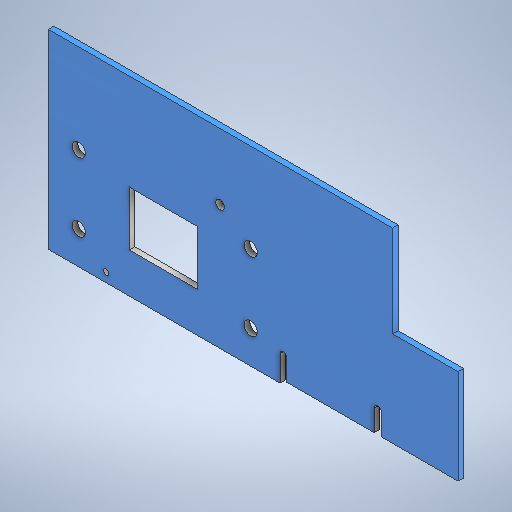
# Autodesk Inventor part: daughterboard
Saved by Autodesk Inventor 2025.1 (Build 291241000, 241)
## iProperties
Created: 2024-09-23
Part Number: daughterboard
Material: Generic
Document SubType Name: Modeling
Designer: PC
Density: 1 g/cm^3
Appearance: Default
Author: PC
Autodesk Inventor part; units mm, degrees
ref_plane "YZ Plane" through (0, 0, 0) normal (1, 0, 0) x (0, 1, 0)
ref_plane "XZ Plane" through (0, 0, 0) normal (0, 1, 0) x (-1, 0, 0)
ref_plane "XY Plane" through (0, 0, 0) normal (0, 0, 1) x (1, 0, 0)
sketch "Sketch1" plane through (0, 0, 0) normal (0, 0, 1) x (1, 0, 0)
  line L0 (0, 0) -> (125, 0)
  line L1 (125, 1.25) -> (125, 30.15)
  line L2 (105, 58.1) -> (0, 58.1)
  line L3 (0, 58.1) -> (0, 0)
  line L4 (105, 58.1) -> (105, 30.15)
  line L5 (105, 30.15) -> (125, 30.15)
  line L6 (24.7, 28.775) -> (45.44, 28.775)
  line L7 (45.44, 28.775) -> (45.44, 12.175)
  line L8 (45.44, 12.175) -> (24.7, 12.175)
  line L9 (24.7, 12.175) -> (24.7, 28.775)
  circle A0 centre (9.3, 10) radius 2
  circle A1 centre (61.75, 10) radius 2
  circle A2 centre (9.3, 30.95) radius 2
  circle A3 centre (61.75, 30.95) radius 2
  line L10 (9.3, 30.95) -> (9.3, 10) construction
  line L11 (9.3, 10) -> (61.75, 10) construction
  line L12 (70.7, 0) -> (70.7, 1.25)
  arc A4 (72.7, 7.8) -> (70.7, 7.8) centre (71.7, 7.8) ccw
  line L13 (70.7, 7.8) -> (70.7, 1.25)
  line L14 (72.7, 7.8) -> (72.7, 1.25)
  arc A5 (101.6, 7.8) -> (99.4, 7.8) centre (100.5, 7.8) ccw
  line L15 (99.4, 7.8) -> (99.4, 1.25)
  line L16 (101.6, 7.8) -> (101.6, 1.25)
  line L17 (72.7, 1.25) -> (99.4, 1.25)
  line L18 (101.6, 1.25) -> (125, 1.25)
  circle A6 centre (52.4, 38) radius 1.3
  circle A7 centre (17.7, 2.8) radius 0.8
  point P0 (35.07, 12.175)
  point P1 (35.525, 10)
  point P2 (9.3, 20.475)
  point P3 (24.7, 20.475)
  dimension "d2" = 20
  dimension "d4" = 125
  dimension "d5" = 20.74
  dimension "d9" = 52.45
  dimension "d12" = 20.95
  dimension "d15" = 10
  dimension "d17" = 4
  dimension "d20" = 7.8
  dimension "d27" = 2.6
  dimension "d28" = 1.6
  dimension "d31" = 16.6
  dimension "d37" = 26.7
  dimension "d40" = 17.7
  dimension "d41" = 9.3
  dimension "d42" = 2.8
  dimension "d43" = 52.4
  dimension "d44" = 38
  dimension "d45" = 24.7
  dimension "d46" = 70.7
  dimension "d47" = 58.1
  dimension "d48" = 2
  dimension "d49" = 2.2
  dimension "d50" = 1.25
  dimension "d52" = 28.9
  constraints: 38 end point, 11 perpendicular, 8 centre point, 5 tangent, 4 coincident, 4 horizontal, 4 midpoint, 4 parallel, 4 point on circle, 3 vertical, 2 horizontal alignment, 1 collinear, 1 point on line, 6 other
  measures "d2" distance of L1.end L4.end
  measures "d4" distance between parallel lines of L3 L1
  measures "d5" distance of L6.start L6.end
  measures "d9" distance of L10.end L11.end
  measures "d12" distance of L10.end L10.start
  measures "d15" distance from line of L0 L10.end
  measures "d17" diameter of A2
  measures "d20" vertical distance of L12.start A4.centre
  measures "d27" diameter of A6
  measures "d28" diameter of A7
  measures "d31" distance of L6.start L8.end
  measures "d37" distance of L14.end L15.end
  measures "d40" distance from line of L3 A7.centre
  measures "d41" distance from line of L3 L10.end
  measures "d42" distance from line of L0 A7.centre
  measures "d43" distance from line of L3 A6.centre
  measures "d44" distance from line of L0 A6.centre
  measures "d45" distance between parallel lines of L3 L9
  measures "d46" distance between parallel lines of L3 L13
  measures "d47" distance between parallel lines of L0 L2
  measures "d48" distance between parallel lines of L13 L14
  measures "d49" distance between parallel lines of L16 L15
  measures "d50" distance between parallel lines of L0 L17
  measures "d52" distance between parallel lines of L18 L5
extrude "Extrusion1" add sketch "Sketch1" along normal blind 1.7
body "Solid1"
